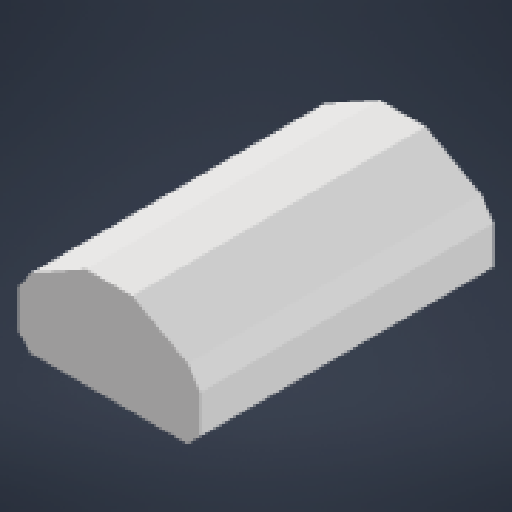
# Autodesk Inventor part: charge_port_plug
Saved by Autodesk Inventor 2026.1 (Build 301233000, 233)
## iProperties
Created: 2026-07-14
Part Number: charge_port_plug
Material: Generic
Document SubType Name: Modeling
Designer: aaron
Density: 1 g/cm^3
Appearance: Default
Author: aaron
Autodesk Inventor part; units mm, degrees
ref_plane "YZ Plane" through (0, 0, 0) normal (1, 0, 0) x (0, 1, 0)
ref_plane "XZ Plane" through (0, 0, 0) normal (0, 1, 0) x (-1, 0, 0)
ref_plane "XY Plane" through (0, 0, 0) normal (0, 0, 1) x (1, 0, 0)
sketch "Sketch1" plane through (0, 0, 0) normal (0, 0, 1) x (1, 0, 0)
  line L0 (-23.7129, 7.994) -> (-21.7129, 5.994)
  line L1 (-21.7129, 0.4463) -> (-21.7129, 5.994)
  line L2 (-19.7129, -1.5537) -> (-21.7129, 0.4463)
  line L3 (3.2871, -1.5537) -> (-19.7129, -1.5537)
  line L4 (5.2871, 0.4463) -> (3.2871, -1.5537)
  line L5 (5.2871, 5.994) -> (5.2871, 0.4463)
  line L6 (5.2871, 5.994) -> (7.2871, 7.994)
  line L7 (-23.5715, 8.1354) -> (-21.5129, 6.0768)
  line L8 (-21.5129, 6.0768) -> (-21.5129, 0.5292)
  line L9 (-21.5129, 0.5292) -> (-19.6301, -1.3537)
  line L10 (-19.6301, -1.3537) -> (3.2042, -1.3537)
  line L11 (3.2042, -1.3537) -> (5.0871, 0.5292)
  line L12 (5.0871, 0.5292) -> (5.0871, 6.0768)
  line L13 (5.0871, 6.0768) -> (7.1456, 8.1354)
  line L14 (-21.5129, 6.0768) -> (-19.6301, 8.8175)
  line L15 (-19.6301, 8.8175) -> (-11.568, 13.3014)
  line L16 (-11.568, 13.3014) -> (-8.2129, 13.3014)
  line L17 (-19.7129, -1.5537) -> (-19.7129, -4.3475)
  line L18 (-19.7129, -4.3475) -> (-8.2129, -4.3475)
  line L19 (-8.2129, -4.3475) -> (-8.2129, 15.1673)
  line L20 (5.0871, 6.0768) -> (3.2042, 8.8175)
  line L21 (3.2042, 8.8175) -> (-4.8579, 13.3014)
  line L22 (-4.8579, 13.3014) -> (-8.2129, 13.3014)
  point P0 (0, 0)
  dimension "d0" = 0.2
  dimension "d1" = 23
  dimension "d2" = 11.5
  constraints: 46 end point, 2 symmetric about line, 2 vertical, 1 horizontal, 1 perpendicular, 1 point on line, 6 other
  measures "d0" distance between parallel lines of L3 L10
  measures "d1" distance of L3.start L2.start
  measures "d2" distance of L17.end L18.end
extrude "Extrusion1" add sketch "Sketch1" along normal blind 42.8 contours L14 L15 L16 L19 L10 L9 L8 | L19 L22 L21 L20 L12 L11 L10
sketch "Sketch2" plane through (0, 0, 0) normal (0, 0, -1) x (-1, 0, 0)
  line L0 (13.2269, 1.874) -> (13.2269, 5.874) projected
  line L1 (3.0769, 5.874) -> (13.2269, 5.874) projected
  line L2 (3.0769, 5.874) -> (3.0769, 1.874) projected
  line L3 (3.6906, 5.9511) -> (12.5906, 5.9511)
  line L4 (12.5906, 5.9511) -> (12.5906, 1.9511)
  line L5 (12.5906, 1.9511) -> (3.6906, 1.9511)
  line L6 (3.6906, 1.9511) -> (3.6906, 5.9511)
  point P0 (0, 0)
  dimension "d5" = 4
  dimension "d6" = 8.9
  constraints: 8 end point, 2 parallel, 1 horizontal, 1 perpendicular
  measures "d5" distance between parallel lines of L3 L5
  measures "d6" distance of L3.start L3.end
extrude "Extrusion2" cut sketch "Sketch2" against normal blind 4.8
sketch "Sketch3" plane through (0, 0, 4.8) normal (0, 0, -1) x (-1, 0, 0)
  line L0 (-8.749, 6.2089) -> (25.106, 6.2089)
  line L1 (25.106, 6.2089) -> (25.106, 1.7089)
  line L2 (25.106, 1.7089) -> (-8.749, 1.7089)
  line L3 (-8.749, 1.7089) -> (-8.749, 6.2089)
  point P0 (0, 0)
  dimension "d9" = 4.5
  constraints: 8 end point, 2 parallel, 1 horizontal, 1 perpendicular
  measures "d9" distance between parallel lines of L0 L2
extrude "Extrusion3" cut sketch "Sketch3" against normal through all
sketch "Sketch4" plane through (-19.6301, -1.3537, 0) normal (0, -1, 0) x (1, 0, 0)
  line L0 (0, 0) -> (0, 42.8) projected
  line L1 (0, 39.8) -> (11.4172, 39.8)
  line L2 (11.4172, 39.8) -> (22.8343, 39.8)
  line L3 (22.8343, 0) -> (22.8343, 42.8) projected
  circle A0 centre (11.4172, 39.8) radius 1.65
  line L4 (0, 42.8) -> (22.8343, 42.8) projected
  point P0 (19.6301, 0)
  dimension "d12" = 3
  dimension "d13" = 3.3
  constraints: 4 end point, 3 point on line, 1 centre point, 1 coincident, 1 collinear, 1 horizontal
  measures "d12" distance between parallel lines of L4 L2
  measures "d13" diameter of A0
extrude "Extrusion4" cut sketch "Sketch4" against normal through all contours A0 L2 L1 | L1 L2 A0
body "Solid1"
